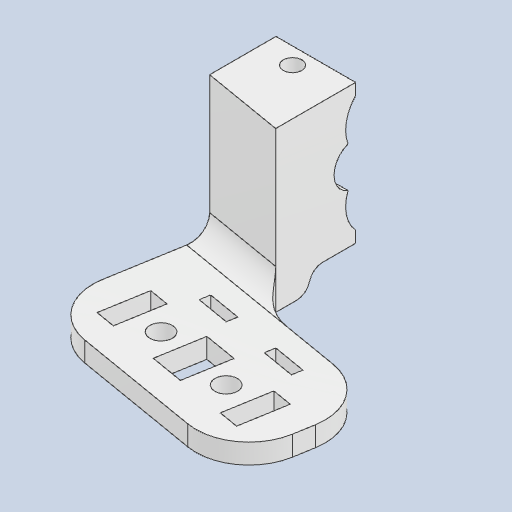
# Autodesk Inventor part: finlay_holds_board2
Saved by Autodesk Inventor 2024 (Build 280153000, 153)
## iProperties
Created: 2024-09-25
Part Number: finlay_holds_board2
Material: ABS プラスチック
Document SubType Name: Modeling
Designer: 1412z
Density: 1.06 g/cm^3
Appearance: 滑らか - 白
Author: 1412z
Autodesk Inventor part; units mm, degrees
ref_plane "YZ Plane" through (0, 0, 0) normal (1, 0, 0) x (0, 1, 0)
ref_plane "XZ Plane" through (0, 0, 0) normal (0, 1, 0) x (-1, 0, 0)
ref_plane "XY Plane" through (0, 0, 0) normal (0, 0, 1) x (1, 0, 0)
sketch "スケッチ1" plane through (0, 0, 0) normal (0, 1, 0) x (-1, 0, 0)
  line L0 (17.5, -12.5) -> (-17.5, -12.5)
  line L1 (-17.5, -12.5) -> (-17.5, 12.5)
  line L2 (-17.5, 12.5) -> (17.5, 12.5)
  line L3 (17.5, 12.5) -> (17.5, -12.5)
  line L4 (17.5, -12.5) -> (-17.5, 12.5) construction
  line L5 (-17.5, -12.5) -> (17.5, 12.5) construction
  point P0 (0, 0)
  dimension "d0" = 35
  dimension "d1" = 25
  constraints: 12 end point, 2 midpoint, 2 parallel, 1 horizontal, 1 perpendicular
  measures "d0" distance of L1.end L2.end
  measures "d1" distance of L0.end L1.end
extrude "押し出し1" add sketch "スケッチ1" along normal mid plane 3
sketch "スケッチ2" plane through (0, 1.5, 0) normal (0, 1, 0) x (1, 0, 0)
  circle A0 centre (6, -5) radius 1.7
  circle A1 centre (-6, -5) radius 1.7
  point P0 (0, 0)
  dimension "d4" = 3.4
  dimension "d5" = 3.4
  constraints: 2 centre point
  measures "d4" diameter of A0
  measures "d5" diameter of A1
extrude "押し出し2" cut sketch "スケッチ2" against normal blind 3
sketch "スケッチ3" plane through (0, 1.5, 0) normal (0, 1, 0) x (1, 0, 0)
  line L0 (2.5, -8.5) -> (-2.5, -8.5)
  line L1 (-2.5, -8.5) -> (-2.5, -1.5)
  line L2 (-2.5, -1.5) -> (2.5, -1.5)
  line L3 (2.5, -1.5) -> (2.5, -8.5)
  line L4 (2.5, -8.5) -> (-2.5, -1.5) construction
  line L5 (-2.5, -8.5) -> (2.5, -1.5) construction
  point P0 (0, 0)
  point P1 (0, -5)
  dimension "d8" = 5
  dimension "d9" = 7
  constraints: 12 end point, 2 midpoint, 2 parallel, 1 horizontal, 1 perpendicular
  measures "d8" distance of L1.end L2.end
  measures "d9" distance of L0.end L1.end
extrude "押し出し3" cut sketch "スケッチ3" against normal blind 3
sketch "スケッチ4" plane through (0, 1.5, 0) normal (0, 1, 0) x (1, 0, 0)
  line L0 (-9.85, -8.5) -> (-12.85, -8.5)
  line L1 (-12.85, -8.5) -> (-12.85, -1.5)
  line L2 (-12.85, -1.5) -> (-9.85, -1.5)
  line L3 (-9.85, -1.5) -> (-9.85, -8.5)
  line L4 (-9.85, -8.5) -> (-12.85, -1.5) construction
  line L5 (-12.85, -8.5) -> (-9.85, -1.5) construction
  line L6 (12.85, -8.5) -> (9.85, -8.5)
  line L7 (9.85, -8.5) -> (9.85, -1.5)
  line L8 (9.85, -1.5) -> (12.85, -1.5)
  line L9 (12.85, -1.5) -> (12.85, -8.5)
  line L10 (12.85, -8.5) -> (9.85, -1.5) construction
  line L11 (9.85, -8.5) -> (12.85, -1.5) construction
  point P0 (0, 0)
  point P1 (-11.35, -5)
  point P2 (11.35, -5)
  dimension "d12" = 3
  dimension "d13" = 7
  dimension "d14" = 3
  dimension "d15" = 7
  constraints: 24 end point, 4 midpoint, 4 parallel, 2 horizontal, 2 perpendicular
  measures "d12" distance of L1.end L2.end
  measures "d13" distance of L0.end L1.end
  measures "d14" distance of L7.end L8.end
  measures "d15" distance of L6.end L7.end
extrude "押し出し4" cut sketch "スケッチ4" against normal blind 3
sketch "スケッチ7" plane through (0, 1.5, 0) normal (0, 1, 0) x (1, 0, 0)
  line L0 (-3.5, 1.75) -> (-8.5, 1.75)
  line L1 (-8.5, 1.75) -> (-8.5, 3.25)
  line L2 (-8.5, 3.25) -> (-3.5, 3.25)
  line L3 (-3.5, 3.25) -> (-3.5, 1.75)
  line L4 (-3.5, 1.75) -> (-8.5, 3.25) construction
  line L5 (-8.5, 1.75) -> (-3.5, 3.25) construction
  line L6 (3.5, 3.25) -> (8.5, 3.25)
  line L7 (8.5, 3.25) -> (8.5, 1.75)
  line L8 (8.5, 1.75) -> (3.5, 1.75)
  line L9 (3.5, 1.75) -> (3.5, 3.25)
  line L10 (3.5, 3.25) -> (8.5, 1.75) construction
  line L11 (8.5, 3.25) -> (3.5, 1.75) construction
  point P0 (0, 0)
  point P1 (-6, 2.5)
  point P2 (6, 2.5)
  dimension "d30" = 5
  dimension "d31" = 1.5
  dimension "d32" = 5
  dimension "d33" = 1.5
  constraints: 24 end point, 4 midpoint, 4 parallel, 2 horizontal, 2 perpendicular
  measures "d30" distance of L1.end L2.end
  measures "d31" distance of L0.end L1.end
  measures "d32" distance of L7.end L8.end
  measures "d33" distance of L6.end L7.end
extrude "押し出し7" cut sketch "スケッチ7" against normal blind 10
sketch "スケッチ15" plane through (17.5, 1.5, -12.5) normal (0, 0, -1) x (-1, 0, 0)
  line L0 (0, -3) -> (0, 0) projected
  line L1 (0, -3) -> (35, -3) projected
  line L2 (0, 0) -> (35, 0)
  line L3 (35, 0) -> (35, -3)
  line L4 (35, -3) -> (0, -3)
  line L5 (0, -3) -> (0, 0)
  point P0 (17.5, -1.5)
  constraints: 8 end point, 2 parallel, 1 horizontal, 1 perpendicular
extrude "押し出し15" cut sketch "スケッチ15" against normal blind 3
sketch "スケッチ16" plane through (0, -1.5, 0) normal (0, -1, 0) x (1, 0, 0)
  line L0 (-17.5, -9.5) -> (-17.5, 12.5) projected
  line L1 (-17.5, -9.5) -> (-19.178, -19.3582)
  line L2 (-17.5, -9.5) -> (-7.5, -9.5) construction
  line L3 (-19.178, -19.3582) -> (15.3257, -25.2313)
  line L4 (-19.178, -19.3582) -> (15.822, -19.3582) construction
  line L5 (17.5, -9.5) -> (17.5, 12.5) projected
  line L6 (15.3257, -25.2313) -> (17.5, -9.5)
  line L7 (-17.5, -9.5) -> (17.5, -9.5) projected
  line L8 (-17.5, -9.5) -> (17.5, -9.5)
  point P0 (0, 0)
  dimension "d64" = 10
  dimension "d65" = 99.66
  dimension "d66" = 35
  dimension "d67" = 9.66
  constraints: 12 end point, 2 equal length, 2 horizontal, 1 collinear
  measures "d64" distance of L0.start L1.end
  measures "d65" angle of L1 L2
  measures "d66" distance of L1.end L3.end
  measures "d67" angle of L3 L4
extrude "押し出し16" add sketch "スケッチ16" against normal blind 27
move or copy body "ボディを移動2" bodies to move or copy 1 copy no rotation origin (0, 0, 0) rotation axis (0, 1, 0) rotation angle -9.66 translate (-3.5203, 0, 2.9436)
sketch "スケッチ17" plane through (-19.178, -1.5, -19.3582) normal (0, -1, 0) x (1, 0, 0)
  circle A0 centre (5, 2.5) radius 1.4
  point P0 (19.178, 19.3582)
  dimension "d71" = 2.8
  constraints: 1 centre point
  measures "d71" diameter of A0
extrude "押し出し17" cut sketch "スケッチ17" against normal blind 27
sketch "スケッチ18" plane through (15.822, -1.5, -19.3582) normal (0, 0, -1) x (-1, 0, 0)
  line L0 (33.7, 13.5) -> (33.7, 5.8)
  line L1 (33.7, 5.8) -> (26.1, 5.8)
  line L2 (26.1, 5.8) -> (26.1, 21.2)
  line L3 (26.1, 21.2) -> (33.7, 21.2)
  line L4 (33.7, 21.2) -> (33.7, 13.5)
  point P0 (15.822, 1.5)
  dimension "d74" = 7.7
  dimension "d75" = 7.6
  dimension "d76" = 15.4
  constraints: 10 end point, 4 perpendicular, 1 point on line, 1 vertical
  measures "d74" distance of L0.start L0.end
  measures "d75" distance of L0.end L1.end
  measures "d76" distance of L1.end L2.end
extrude "押し出し18" cut sketch "スケッチ18" against normal blind 5
sketch "スケッチ19" plane through (-19.178, -1.5, -19.3582) normal (-1, 0, 0) x (0, 0, 1)
  line L0 (0, 21.2) -> (0, 5.8) projected
  circle A0 centre (0, 13.5) radius 3.25
  point P0 (19.3582, 1.5)
  point P1 (0, 16.75)
  point P2 (0, 10.25)
  dimension "d79" = 6.5
  constraints: 1 centre point, 1 midpoint
  measures "d79" diameter of A0
extrude "押し出し19" cut sketch "スケッチ19" against normal blind 40 contours A0 L0 picked at (0.47, 14.476)
sketch "スケッチ20" plane through (-19.178, -1.5, -19.3582) normal (0, -1, 0) x (1, 0, 0)
  line L0 (35, 0) -> (0, 0) projected
  line L1 (12, 0) -> (12, 12.0426)
  line L2 (0, 10) -> (34.5037, 15.873) projected
  line L3 (35, 0) -> (34.5037, 15.873) projected
  line L4 (12, 12.0426) -> (34.5037, 15.873)
  line L5 (34.5037, 15.873) -> (35, 0)
  line L6 (35, 0) -> (12, 0)
  point P0 (19.178, 19.3582)
  constraints: 8 end point, 2 point on line, 1 collinear, 1 perpendicular, 1 vertical
extrude "押し出し20" cut sketch "スケッチ20" against normal blind 40
sketch "スケッチ21" plane through (-19.178, -1.5, -19.3582) normal (0, -1, 0) x (1, 0, 0)
  line L0 (1.3, 0) -> (0, 0) projected
  line L1 (0, 0) -> (0, 7)
  line L2 (0, 10) -> (0, 0) projected
  line L3 (0, 7) -> (12, 7)
  line L4 (12, 12.0426) -> (12, 0) projected
  line L5 (12, 7) -> (12, 0)
  line L6 (12, 0) -> (0, 0)
  point P0 (19.178, 19.3582)
  dimension "d85" = 7
  constraints: 8 end point, 2 perpendicular, 2 point on line, 1 vertical
  measures "d85" distance of L0.end L1.end
extrude "押し出し21" cut sketch "スケッチ21" against normal blind 3
sketch "スケッチ22" plane through (-19.178, 25.5, -9.3582) normal (0, 1, 0) x (1, 0, 0)
  line L0 (0, 10) -> (1.3, 10) projected
  line L1 (0, 0) -> (0, 3) projected
  line L2 (0, 10) -> (0, 0)
  line L3 (12, -2.0426) -> (12, -0.3542) projected
  line L4 (0, 0) -> (12, -2.0426)
  line L5 (12, -2.0426) -> (12, 10)
  line L6 (12, 10) -> (0, 10)
  point P0 (19.178, -9.3582)
  constraints: 8 end point, 1 collinear, 1 parallel, 1 perpendicular
extrude "押し出し22" cut sketch "スケッチ22" against normal blind 3
fillet "フィレット3" radius 2 2 edges at (-13.178, 1.5, -12.3582) (-13.178, -1.5, -12.3582)
sketch "スケッチ23" plane through (-7.178, 12, -19.3582) normal (1, 0, 0) x (0, 0, -1)
  circle A0 centre (4, 5) radius 5.5
  circle A1 centre (4, -5) radius 5.5
  point P0 (-19.3582, -12)
  point P1 (1.7087, 0)
  point P2 (6.2913, 0)
  dimension "d92" = 11
  dimension "d93" = 11
  constraints: 2 centre point
  measures "d92" diameter of A0
  measures "d93" diameter of A1
extrude "押し出し23" cut sketch "スケッチ23" against normal blind 40 contours A0 A1 | A0 A1 picked at (4.0884, 7.1397) picked at (4.0884, -7.1397)
sketch "スケッチ24" plane through (15.3257, -1.5, -3.4852) normal (0.1678012, 0, -0.9858209) x (-0.9858209, 0, -0.1678012)
  line L0 (0, 0) -> (35, 0) projected
  line L1 (22.8274, 0) -> (22.8274, 3) projected
  line L2 (0, 0) -> (22.8274, 0)
  line L3 (22.8274, 0) -> (22.8274, 3)
  line L4 (26, 3) -> (21, 3) projected
  line L5 (0, 0) -> (0, 3) projected
  line L6 (0, 0) -> (0, 3)
  line L7 (0, 3) -> (22.8274, 3)
  point P0 (14.5236, 1.5)
  point P1 (21, 3)
  constraints: 8 end point, 3 perpendicular, 1 collinear, 1 point on line
extrude "押し出し24" cut sketch "スケッチ24" against normal blind 3
fillet "フィレット5" radius 8 4 edges at (14.822, 0, -0.5257) (-7.6818, 0, -4.3562) (-22.8696, 0, 12.3299) (11.6341, 0, 18.2029)
fillet "フィレット6" radius 3 1 edges at (-13.178, 1.5, -8.3369)
